Autodesk Inventor part; units mm, degrees
(part 2 of 2)
  spline S298 degree 2 poles (-159.8121, 51.7816) (-160.0049, 51.6827) (-160.2224, 51.3515) (-160.2421, 51.1043) knots 0 0 0 1 2 2 2
  line L81 (-160.2421, 51.1043) -> (-161.5768, 51.1043)
  line L82 (-161.5768, 51.1043) -> (-161.5768, 56.1563)
  line L83 (-161.5768, 56.1563) -> (-162.8324, 56.1563)
  line L84 (-162.8324, 56.1563) -> (-162.8324, 57.2192)
  spline S299 degree 2 poles (-168.2898, 53.8281) (-168.2898, 54.6042) (-167.9289, 55.8993) (-167.5483, 56.364) knots 0 0 0 1 2 2 2
  spline S300 degree 2 poles (-167.5483, 56.364) (-167.1528, 56.8336) (-165.9862, 57.3378) (-165.136, 57.3378) knots 0 0 0 1 2 2 2
  spline S301 degree 2 poles (-165.136, 57.3378) (-164.8493, 57.3378) (-164.2264, 57.2636) (-164.1226, 57.234) knots 0 0 0 1 2 2 2
  line L85 (-164.1226, 57.234) -> (-164.1226, 56.0377)
  line L86 (-164.1226, 56.0377) -> (-164.2412, 56.0377)
  spline S302 degree 2 poles (-164.2412, 56.0377) (-164.3549, 56.097) (-164.7801, 56.2256) (-165.1508, 56.2256) knots 0 0 0 1 2 2 2
  spline S303 degree 2 poles (-165.1508, 56.2256) (-165.4524, 56.2256) (-166.0109, 56.0674) (-166.2087, 55.8944) knots 0 0 0 1 2 2 2
  spline S304 degree 2 poles (-166.2087, 55.8944) (-166.4212, 55.7115) (-166.6981, 55.1726) (-166.7475, 54.7673) knots 0 0 0 1 2 2 2
  spline S305 degree 2 poles (-166.7475, 54.7673) (-166.4212, 54.97) (-165.8577, 55.1875) (-165.4375, 55.1875) knots 0 0 0 1 2 2 2
  spline S306 degree 2 poles (-165.4375, 55.1875) (-165.1261, 55.1875) (-164.5477, 55.0194) (-164.3105, 54.8414) knots 0 0 0 1 2 2 2
  spline S307 degree 2 poles (-164.3105, 54.8414) (-163.9941, 54.5992) (-163.6233, 53.8231) (-163.6233, 53.2102) knots 0 0 0 1 2 2 2
  spline S308 degree 2 poles (-163.6233, 53.2102) (-163.6233, 52.7307) (-163.9496, 51.9249) (-164.2462, 51.6283) knots 0 0 0 1 2 2 2
  spline S309 degree 2 poles (-164.2462, 51.6283) (-164.5428, 51.3317) (-165.4029, 50.9956) (-165.9318, 50.9956) knots 0 0 0 1 2 2 2
  spline S310 degree 2 poles (-165.9318, 50.9956) (-166.4657, 50.9956) (-167.2912, 51.2922) (-167.5878, 51.6036) knots 0 0 0 1 2 2 2
  spline S311 degree 2 poles (-167.5878, 51.6036) (-167.9339, 51.9496) (-168.2898, 53.047) (-168.2898, 53.8281) knots 0 0 0 1 2 2 2
  spline S312 degree 2 poles (-166.7722, 53.6007) (-166.7722, 53.1014) (-166.6041, 52.4588) (-166.4509, 52.2808) knots 0 0 0 1 2 2 2
  spline S313 degree 2 poles (-166.4509, 52.2808) (-166.3471, 52.1474) (-166.0801, 52.0337) (-165.9269, 52.0337) knots 0 0 0 1 2 2 2
  spline S314 degree 2 poles (-165.9269, 52.0337) (-165.7885, 52.0337) (-165.5314, 52.1424) (-165.4128, 52.2808) knots 0 0 0 1 2 2 2
  spline S315 degree 2 poles (-165.4128, 52.2808) (-165.309, 52.3995) (-165.1607, 52.8592) (-165.1607, 53.1311) knots 0 0 0 1 2 2 2
  spline S316 degree 2 poles (-165.1607, 53.1311) (-165.1607, 53.4277) (-165.3139, 53.8083) (-165.4425, 53.922) knots 0 0 0 1 2 2 2
  spline S317 degree 2 poles (-165.4425, 53.922) (-165.5759, 54.0357) (-165.9071, 54.1247) (-166.1147, 54.1247) knots 0 0 0 1 2 2 2
  spline S318 degree 2 poles (-166.1147, 54.1247) (-166.2878, 54.1247) (-166.6486, 54.0307) (-166.7623, 53.9813) knots 0 0 0 1 2 2 2
  spline S319 degree 2 poles (-166.7623, 53.9813) (-166.7623, 53.9368) (-166.7722, 53.7687) (-166.7722, 53.6007) knots 0 0 0 1 2 2 2
  point P0 (-85, 53)
  dimension "d42" = 18
  dimension "d43" = 5
  dimension "d44" = 5
  dimension "d45" = 5
  dimension "d46" = 5
  dimension "d47" = 5
  dimension "d49" = 10
  dimension "d50" = 10
  dimension "d51" = 20
  dimension "d52" = 20
  dimension "d53" = 5
  dimension "d54" = 5
  dimension "d55" = 5
  dimension "d56" = 5
  dimension "d62" = 1
  dimension "d63" = 1
  dimension "d64" = 1
  constraints: 33 end point, 16 point on circle, 16 tangent, 15 point on line, 8 centre point, 8 perpendicular, 5 collinear, 2 horizontal, 1 equal radius, 6 other
  measures "d42" distance between parallel lines of L5 L4
  measures "d43" distance between parallel lines of L2 L9
  measures "d44" distance of L6.end L7.end
  measures "d45" distance of L10.end L11.end
  measures "d46" distance of L16.start L13.start
  measures "d47" distance of L14.end L15.end
  measures "d49" distance of point (-152, 7.317) L6.end
  measures "d50" distance of L13.start point (-18, 7.317)
  measures "d51" distance between parallel lines of L14 L13
  measures "d52" distance between parallel lines of L12 L6
  measures "d53" radius of A0
  measures "d54" radius of A1
  measures "d55" radius of A2
  measures "d56" radius of A3
  measures "d62" radius of A4
  measures "d63" radius of A5
  measures "d64" radius of A6
sketch "Sketch3" plane through (-22, -53, 85) normal (-1, 0, 0) x (0, 0, 1)
  point P0 (-85, 53)
extrude "Extrusion7" cut sketch "Sketch2" against normal blind 4
body "Solid1"
